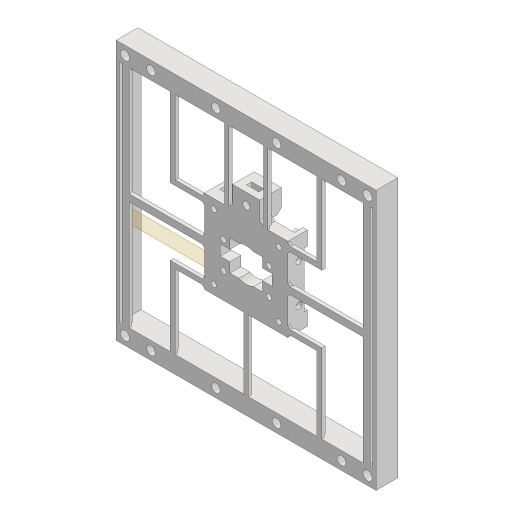
# Autodesk Inventor part: Flexible_cam_holder_v7_HQ
Saved by Autodesk Inventor 2023 (Build 270158000, 158)
## iProperties
Created: 2021-01-08
Part Number: Flexible_cam_holder_v7_HQ
Material: Generic
Document SubType Name: Sheet Metal
Designer: CDT
Density: 1 g/cm^3
Appearance: Default
Sheet Metal Rule: Default
Author: CDT
Autodesk Inventor part; units mm, degrees
ref_plane "YZ Plane" through (0, 0, 0) normal (1, 0, 0) x (0, 1, 0)
ref_plane "XZ Plane" through (0, 0, 0) normal (0, 1, 0) x (-1, 0, 0)
ref_plane "Work Plane1" through (0, 0, 0) normal (0, 0, 1) x (1, 0, 0)
sketch "Sketch1" plane through (0, 0, 0) normal (0, 0, 1) x (1, 0, 0)
  line L0 (-30.0874, -48.0547) -> (89.9126, -48.0547)
  line L1 (89.9126, -48.0547) -> (89.9126, 71.9453)
  line L2 (89.9126, 71.9453) -> (-30.0874, 71.9453)
  line L3 (-30.0874, 71.9453) -> (-30.0874, -48.0547)
  circle A0 centre (-26.0874, 67.9453) radius 2.125
  circle A1 centre (85.9126, 67.9453) radius 2.125
  circle A2 centre (85.9126, -44.0547) radius 2.125
  circle A3 centre (-26.0874, -44.0547) radius 2.125
  circle A4 centre (-14.0874, 67.9453) radius 2
  circle A5 centre (73.9126, 67.9453) radius 2
  circle A6 centre (-14.0874, -44.0547) radius 2
  circle A7 centre (73.9126, -44.0547) radius 2
  circle A8 centre (15.9126, 67.9453) radius 2
  circle A9 centre (43.9126, 67.9453) radius 2
  circle A10 centre (15.9126, -44.0547) radius 2
  circle A11 centre (43.9126, -44.0547) radius 2
  point P0 (0, 0)
  dimension "d0" = 120
  dimension "d1" = 120
  dimension "d2" = 4.25
  dimension "d3" = 4.25
  dimension "d4" = 4.25
  dimension "d5" = 4.25
  dimension "d107" = 4
  dimension "d108" = 4
  dimension "d109" = 4
  dimension "d110" = 4
  dimension "d111" = 4
  dimension "d112" = 4
  dimension "d113" = 4
  dimension "d114" = 4
  dimension "d172" = 4
  dimension "d173" = 4
  dimension "d174" = 4
  dimension "d175" = 4
  dimension "d176" = 16
  dimension "d177" = 4
  dimension "d178" = 4
  dimension "d179" = 16
  dimension "d180" = 16
  dimension "d181" = 4
  dimension "d182" = 4
  dimension "d183" = 16
  dimension "d729" = 4
  dimension "d730" = 4
  dimension "d731" = 4
  dimension "d732" = 4
  dimension "d733" = 4
  dimension "d734" = 4
  dimension "d735" = 4
  dimension "d736" = 4
  dimension "d737" = 46
  dimension "d738" = 46
  dimension "d739" = 46
  dimension "d740" = 46
  constraints: 12 centre point, 8 end point, 2 parallel, 1 horizontal, 1 perpendicular
  measures "d0" distance of L2.end L0.start
  measures "d1" distance of L1.end L2.end
  measures "d2" diameter of A0
  measures "d3" diameter of A1
  measures "d4" diameter of A2
  measures "d5" diameter of A3
  measures "d107" distance from line of L1 A1.centre
  measures "d108" distance from line of L3 A0.centre
  measures "d109" distance from line of L3 A3.centre
  measures "d110" distance from line of L1 A2.centre
  measures "d111" distance from line of L2 A0.centre
  measures "d112" distance from line of L2 A1.centre
  measures "d113" distance from line of L0 A2.centre
  measures "d114" distance from line of L0 A3.centre
  measures "d172" diameter of A4
  measures "d173" diameter of A5
  measures "d174" diameter of A6
  measures "d175" diameter of A7
  measures "d176" distance from line of A6.centre L3
  measures "d177" distance from line of L0 A6.centre
  measures "d178" distance from line of L0 A7.centre
  measures "d179" distance from line of L1 A7.centre
  measures "d180" distance from line of L1 A5.centre
  measures "d181" distance from line of L2 A5.centre
  measures "d182" distance from line of L2 A4.centre
  measures "d183" distance from line of L3 A4.centre
  measures "d729" diameter of A8
  measures "d730" diameter of A9
  measures "d731" diameter of A10
  measures "d732" diameter of A11
  measures "d733" distance from line of L2 A9.centre
  measures "d734" distance from line of L2 A8.centre
  measures "d735" distance from line of L0 A10.centre
  measures "d736" distance from line of L0 A11.centre
  measures "d737" distance from line of L1 A11.centre
  measures "d738" distance from line of L3 A10.centre
  measures "d739" distance from line of L3 A8.centre
  measures "d740" distance from line of L1 A9.centre
extrude "Extrusion1" add sketch "Sketch1" along normal blind 5
sketch "Sketch2" plane through (0, 0, 5) normal (0, 0, 1) x (1, 0, 0)
  line L0 (-24.0874, -40.0547) -> (10.6626, -40.0547)
  line L1 (10.6626, -40.0547) -> (10.6626, 10.3453)
  line L2 (10.6626, 10.3453) -> (-24.0874, 10.3453)
  line L3 (-24.0874, 10.3453) -> (-24.0874, -40.0547)
  line L4 (89.9126, -48.0547) -> (89.9126, 71.9453) projected
  line L5 (-30.0874, 71.9453) -> (-30.0874, -48.0547) projected
  line L6 (-30.0874, -48.0547) -> (89.9126, -48.0547) projected
  line L7 (89.9126, 71.9453) -> (-30.0874, 71.9453) projected
  line L8 (-24.0874, 13.5453) -> (10.6626, 13.5453)
  line L9 (10.6626, 13.5453) -> (10.6626, 63.9453)
  line L10 (10.6626, 63.9453) -> (-24.0874, 63.9453)
  line L11 (-24.0874, 63.9453) -> (-24.0874, 13.5453)
  line L12 (83.9126, -40.0547) -> (49.1626, -40.0547)
  line L13 (49.1626, -40.0547) -> (49.1626, 10.3453)
  line L14 (49.1626, 10.3453) -> (83.9126, 10.3453)
  line L15 (83.9126, 10.3453) -> (83.9126, -40.0547)
  line L16 (83.9126, 13.5453) -> (49.1626, 13.5453)
  line L17 (49.1626, 13.5453) -> (49.1626, 63.9453)
  line L18 (49.1626, 63.9453) -> (83.9126, 63.9453)
  line L19 (83.9126, 63.9453) -> (83.9126, 13.5453)
  line L20 (-24.0874, -40.0547) -> (83.9126, -40.0547)
  line L21 (83.9126, -40.0547) -> (83.9126, -7.3047)
  line L22 (83.9126, -7.3047) -> (-24.0874, -7.3047)
  line L23 (-24.0874, -7.3047) -> (-24.0874, -40.0547)
  line L24 (-24.0874, 63.9453) -> (83.9126, 63.9453)
  line L25 (83.9126, 63.9453) -> (83.9126, 31.1953)
  line L26 (83.9126, 31.1953) -> (-24.0874, 31.1953)
  line L27 (-24.0874, 31.1953) -> (-24.0874, 63.9453)
  line L28 (83.9126, 11.9453) -> (49.1626, 11.9453)
  line L29 (49.1626, 11.9453) -> (49.1626, 11.9453)
  line L30 (49.1626, 11.9453) -> (83.9126, 11.9453)
  line L31 (83.9126, 11.9453) -> (83.9126, 11.9453)
  line L32 (15.6626, 11.9453) -> (-24.0874, 11.9453)
  line L33 (-24.0874, 11.9453) -> (-24.0874, 11.9453)
  line L34 (-24.0874, 11.9453) -> (15.6626, 11.9453)
  line L35 (15.6626, 11.9453) -> (15.6626, 11.9453)
  line L36 (-27.3874, -40.0547) -> (-30.0874, -40.0547)
  line L37 (-30.0874, -40.0547) -> (-30.0874, 63.9453)
  line L38 (-30.0874, 63.9453) -> (-27.3874, 63.9453)
  line L39 (-27.3874, 63.9453) -> (-27.3874, -40.0547)
  line L40 (89.9126, 63.9453) -> (87.2126, 63.9453)
  line L41 (87.2126, 63.9453) -> (87.2126, -40.0547)
  line L42 (87.2126, -40.0547) -> (89.9126, -40.0547)
  line L43 (89.9126, -40.0547) -> (89.9126, 63.9453)
  line L44 (-30.0874, -48.0547) -> (-44.0088, -48.0547)
  line L45 (-44.0088, -48.0547) -> (-44.0088, 71.9453)
  line L46 (-44.0088, 71.9453) -> (-30.0874, 71.9453)
  line L47 (-30.0874, 71.9453) -> (-30.0874, -48.0547)
  point P0 (0, 0)
  point P1 (10.6626, 63.9453)
  point P2 (10.6626, 31.1953)
  point P3 (49.1626, 31.1953)
  point P4 (49.1626, -7.3047)
  point P5 (10.6626, -7.3047)
  point P6 (10.6626, -40.0547)
  point P7 (-30.0874, 63.9453)
  point P8 (-30.0874, -40.0547)
  point P9 (89.9126, -40.0547)
  dimension "d9" = 6
  dimension "d10" = 8
  dimension "d13" = 8
  dimension "d15" = 6
  dimension "d19" = 6
  dimension "d20" = 6
  dimension "d21" = 8
  dimension "d23" = 6
  dimension "d24" = 58.4
  dimension "d25" = 58.4
  dimension "d26" = 32.75
  dimension "d27" = 32.75
  dimension "d31" = 58.4
  dimension "d32" = 58.4
  dimension "d54" = 1.6
  dimension "d55" = 1.6
  dimension "d56" = 6
  dimension "d58" = 6
  dimension "d91" = 0
  dimension "d115" = 8
  dimension "d116" = 8
  dimension "d117" = 3.3
  dimension "d119" = 8
  dimension "d120" = 8
  dimension "d121" = 3.3
  dimension "d168" = 38.5
  dimension "d342" = 120
  dimension "d352" = 120
  dimension "d778" = 38.5
  dimension "d779" = 38.5
  dimension "d780" = 34.75
  dimension "d781" = 34.75
  constraints: 88 end point, 22 equal length, 11 horizontal, 11 perpendicular, 5 point on line, 3 collinear
  measures "d9" distance between parallel lines of L5 L3
  measures "d10" distance between parallel lines of L6 L0
  measures "d13" distance between parallel lines of L7 L10
  measures "d15" distance between parallel lines of L5 L11
  measures "d19" distance between parallel lines of L21 L4
  measures "d20" distance between parallel lines of L4 L15
  measures "d21" distance between parallel lines of L6 L12
  measures "d23" distance between parallel lines of L4 L19
  measures "d24" distance between parallel lines of L6 L14
  measures "d25" distance between parallel lines of L16 L7
  measures "d26" distance between parallel lines of L26 L24
  measures "d27" distance between parallel lines of L22 L20
  measures "d31" distance between parallel lines of L6 L2
  measures "d32" distance between parallel lines of L8 L7
  measures "d54" distance between parallel lines of L14 L28
  measures "d55" distance between parallel lines of L16 L30
  measures "d56" distance between parallel lines of L4 L31
  measures "d58" distance between parallel lines of L5 L33
  measures "d91" distance between parallel lines of L32 L34
  measures "d115" distance between parallel lines of L6 L36
  measures "d116" distance between parallel lines of L7 L38
  measures "d117" distance between parallel lines of L11 L39
  measures "d119" distance between parallel lines of L7 L40
  measures "d120" distance between parallel lines of L6 L42
  measures "d121" distance between parallel lines of L19 L41
  measures "d168" distance between parallel lines of L26 L22
  measures "d342" distance of L4.end L5.start
  measures "d352" distance of L44.end L45.end
  measures "d778" distance between parallel lines of L13 L1
  measures "d779" distance between parallel lines of L17 L9
  measures "d780" distance between parallel lines of L17 L19
  measures "d781" distance between parallel lines of L3 L1
extrude "Extrusion2" cut sketch "Sketch2" against normal blind 10 contours L3 L22 L1 L0 | L1 L22 L13 L20 | L3 L2 L1 L22 | L13 L22 L15 L12 | L13 L14 L15 L22 | L42 L41 L40 L4 | L5 L38 L39 L36 | L11 L26 L9 L8 | L11 L10 L9 L26 | L9 L24 L17 L26 | L26 L19 L16 L17 | L17 L18 L19 L26
sketch "Sketch3" plane through (0, 0, 5) normal (0, 0, 1) x (1, 0, 0)
  circle A0 centre (19.4126, 4.5953) radius 1.25
  circle A1 centre (19.4126, 17.0953) radius 1.25
  circle A2 centre (40.4126, 4.5953) radius 1.25
  circle A3 centre (40.4126, 17.0953) radius 1.25
  line L0 (49.1626, 31.1953) -> (10.6626, 31.1953) projected
  line L1 (10.6626, -7.3047) -> (49.1626, -7.3047) projected
  line L2 (49.1626, -7.3047) -> (49.1626, 10.3453) projected
  line L3 (10.6626, -7.3047) -> (10.6626, 10.3453) projected
  point P0 (0, 0)
  point P1 (36.9126, 39.9453)
  dimension "d257" = 2.5
  dimension "d258" = 2.5
  dimension "d259" = 2.5
  dimension "d260" = 2.5
  dimension "d261" = 12.5
  dimension "d262" = 12.5
  dimension "d263" = 21
  dimension "d264" = 21
  dimension "d265" = 0
  dimension "d266" = 0
  dimension "d455" = 38.5
  dimension "d456" = 38.5
  dimension "d457" = 11.9
  dimension "d458" = 11.9
  dimension "d459" = 8.75
  dimension "d741" = 8.75
  dimension "d759" = 14.1
  constraints: 4 centre point
  measures "d257" diameter of A0
  measures "d258" diameter of A1
  measures "d259" diameter of A2
  measures "d260" diameter of A3
  measures "d261" distance of A3.centre A2.centre
  measures "d262" distance of A1.centre A0.centre
  measures "d263" distance of A3.centre A1.centre
  measures "d264" distance of A2.centre A0.centre
  measures "d265" vertical distance of A2.centre A0.centre
  measures "d266" horizontal distance of A2.centre A3.centre
  measures "d455" distance between parallel lines of L0 L1
  measures "d456" distance of L1.start L1.end
  measures "d457" distance from line of A0.centre L1
  measures "d458" distance from line of L1 A2.centre
  measures "d459" distance from line of L2 A2.centre
  measures "d741" distance from line of L3 A0.centre
  measures "d759" distance from line of L0 A1.centre
ref_plane "Work Plane2" through (-30, 66, 0) normal (0, 0, 1) x (1, 0, 0)
extrude "Extrusion3" cut sketch "Sketch3" against normal up to surface (5 mm away)
sketch "Sketch34" plane through (0, 0, 5) normal (0, 0, 1) x (1, 0, 0)
  line L0 (-5.0874, 63.9453) -> (-2.7874, 63.9453)
  line L1 (-2.7874, 63.9453) -> (-2.7874, 27.4453)
  line L2 (-2.7874, 27.4453) -> (-5.0874, 27.4453)
  line L3 (-5.0874, 27.4453) -> (-5.0874, 63.9453)
  line L4 (-24.0874, 63.9453) -> (83.9126, 63.9453) projected
  line L5 (-24.0874, 13.5453) -> (-24.0874, 63.9453) projected
  line L6 (62.6126, 63.9453) -> (64.9126, 63.9453)
  line L7 (64.9126, 63.9453) -> (64.9126, 27.4453)
  line L8 (64.9126, 27.4453) -> (62.6126, 27.4453)
  line L9 (62.6126, 27.4453) -> (62.6126, 63.9453)
  line L10 (83.9126, 63.9453) -> (83.9126, 13.5453) projected
  line L11 (-2.7874, 27.4453) -> (10.6626, 27.4453)
  line L12 (10.6626, 27.4453) -> (10.6626, 29.7453)
  line L13 (10.6626, 29.7453) -> (-2.7874, 29.7453)
  line L14 (-2.7874, 29.7453) -> (-2.7874, 27.4453)
  line L15 (62.6126, 27.4453) -> (49.1626, 27.4453)
  line L16 (49.1626, 27.4453) -> (49.1626, 29.7453)
  line L17 (49.1626, 29.7453) -> (62.6126, 29.7453)
  line L18 (62.6126, 29.7453) -> (62.6126, 27.4453)
  line L19 (-5.0874, -40.0547) -> (-2.7874, -40.0547)
  line L20 (-2.7874, -40.0547) -> (-2.7874, -3.5547)
  line L21 (-2.7874, -3.5547) -> (-5.0874, -3.5547)
  line L22 (-5.0874, -3.5547) -> (-5.0874, -40.0547)
  line L23 (62.6126, -40.0547) -> (64.9126, -40.0547)
  line L24 (64.9126, -40.0547) -> (64.9126, -3.5547)
  line L25 (64.9126, -3.5547) -> (62.6126, -3.5547)
  line L26 (62.6126, -3.5547) -> (62.6126, -40.0547)
  line L27 (-24.0874, -40.0547) -> (-24.0874, 10.3453) projected
  line L28 (-2.7874, -3.5547) -> (10.6626, -3.5547)
  line L29 (10.6626, -3.5547) -> (10.6626, -5.8547)
  line L30 (10.6626, -5.8547) -> (-2.7874, -5.8547)
  line L31 (-2.7874, -5.8547) -> (-2.7874, -3.5547)
  line L32 (83.9126, 10.3453) -> (83.9126, -40.0547) projected
  line L33 (62.6126, -3.5547) -> (49.1626, -3.5547)
  line L34 (49.1626, -3.5547) -> (49.1626, -5.8547)
  line L35 (49.1626, -5.8547) -> (62.6126, -5.8547)
  line L36 (62.6126, -5.8547) -> (62.6126, -3.5547)
  line L37 (-30.0874, -48.0547) -> (89.9126, -48.0547) projected
  line L38 (89.9126, -48.0547) -> (-30.0874, -48.0547)
  line L39 (-30.0874, -48.0547) -> (-30.0874, -57.7562)
  line L40 (-30.0874, -57.7562) -> (89.9126, -57.7562)
  line L41 (89.9126, -57.7562) -> (89.9126, -48.0547)
  line L42 (-30.0874, 71.9453) -> (-30.0874, -48.0547) projected
  line L43 (-30.0874, -48.0547) -> (-47.0069, -48.0547)
  line L44 (-47.0069, -48.0547) -> (-47.0069, 71.9453)
  line L45 (-47.0069, 71.9453) -> (-30.0874, 71.9453)
  line L46 (-30.0874, 71.9453) -> (-30.0874, -48.0547)
  line L47 (-30.0874, 71.9453) -> (-30.0874, -48.0547) projected
  line L48 (89.9126, 71.9453) -> (-30.0874, 71.9453) projected
  line L49 (-22.0874, -40.0547) -> (81.9126, -40.0547) projected
  line L50 (49.1626, 31.1953) -> (49.1626, 13.5453) projected
  line L51 (49.1626, 10.3453) -> (49.1626, -7.3047) projected
  line L52 (10.6626, 10.3453) -> (10.6626, -7.3047) projected
  line L53 (10.6626, 31.1953) -> (10.6626, 13.5453) projected
  point P0 (-24.0874, 10.3453)
  point P1 (62.6126, -5.8547)
  point P2 (64.9126, 63.9453)
  point P3 (-2.7874, 29.7453)
  point P4 (-2.7874, -5.8547)
  point P5 (-30.0874, -40.0547)
  point P6 (99.9126, -40.0547)
  point P7 (54.1626, 36.1953)
  point P8 (83.9126, -40.0547)
  dimension "d317" = 0
  dimension "d318" = 36.5
  dimension "d319" = 19
  dimension "d320" = 2.3
  dimension "d321" = 2.3
  dimension "d322" = 36.5
  dimension "d323" = 0
  dimension "d324" = 19
  dimension "d326" = 2.3
  dimension "d328" = 2.3
  dimension "d329" = 19
  dimension "d330" = 2.3
  dimension "d333" = 2.3
  dimension "d335" = 19
  dimension "d336" = 2.3
  dimension "d337" = 36.5
  dimension "d339" = 2.3
  dimension "d364" = 120
  dimension "d365" = 120
  dimension "d373" = 36.5
  dimension "d374" = 36.5
  dimension "d782" = 0
  dimension "d783" = 0
  dimension "d785" = 0
  dimension "d786" = 0
  constraints: 80 end point, 20 parallel, 10 horizontal, 10 perpendicular, 2 collinear, 2 other
  measures "d317" distance between parallel lines of L4 L0
  measures "d318" distance between parallel lines of L2 L0
  measures "d319" distance between parallel lines of L3 L5
  measures "d320" distance between parallel lines of L1 L3
  measures "d321" distance of L7.end L8.end
  measures "d322" distance of L6.end L7.end
  measures "d323" distance between parallel lines of L4 L6
  measures "d324" distance between parallel lines of L10 L7
  measures "d326" distance of L12.end L11.end
  measures "d328" distance of L15.end L16.end
  measures "d330" distance between parallel lines of L20 L22
  measures "d333" distance of L28.end L29.end
  measures "d336" distance between parallel lines of L26 L24
  measures "d337" distance between parallel lines of L25 L23
  measures "d339" distance of L34.end L33.end
  measures "d364" distance of L42.start L37.start
  measures "d365" distance of L39.end L40.end
  measures "d373" distance between parallel lines of L49 L28
  measures "d374" distance between parallel lines of L49 L33
  measures "d782" distance between parallel lines of L50 L16
  measures "d783" distance between parallel lines of L51 L34
  measures "d785" distance between parallel lines of L52 L29
  measures "d786" distance between parallel lines of L53 L12
extrude "Extrusion32" add sketch "Sketch34" against normal blind 1.5 contours L0 L1 L2 L3 | L13 L12 L11 L1 | L4 L7 L8 L9 | L9 L15 L16 L17 | L22 L21 L20 L19 | L20 L28 L29 L30 | L26 L25 L24 L23 | L35 L34 L33 L26
chamfer "Chamfer5" distance 1 angle 45 12 edges at (49.1626, 10.3453, 2.5) (10.6626, 10.3453, 2.5) (10.6626, -5.8547, 4.25) (10.6626, -3.5547, 4.25) (49.1626, -3.5547, 4.25) (49.1626, -5.8547, 4.25) (49.1626, 13.5453, 2.5) (49.1626, 27.4453, 4.25) (49.1626, 29.7453, 4.25) (10.6626, 13.5453, 2.5) (10.6626, 27.4453, 4.25) (10.6626, 29.7453, 4.25)
sketch "Sketch38" plane through (0, 0, 0) normal (0, 0, -1) x (-1, 0, 0)
  line L0 (-89.9126, -48.0547) -> (30.0874, -48.0547)
  line L1 (30.0874, -48.0547) -> (30.0874, -40.0547)
  line L2 (30.0874, -40.0547) -> (-89.9126, -40.0547)
  line L3 (-89.9126, -40.0547) -> (-89.9126, -48.0547)
  circle A0 centre (-85.9126, -44.0547) radius 2.125 projected
  circle A1 centre (-85.9126, -44.0547) radius 2.125
  circle A2 centre (-73.9126, -44.0547) radius 2 projected
  circle A3 centre (-73.9126, -44.0547) radius 2
  circle A4 centre (14.0874, -44.0547) radius 2 projected
  circle A5 centre (14.0874, -44.0547) radius 2
  circle A6 centre (26.0874, -44.0547) radius 2.125 projected
  circle A7 centre (26.0874, -44.0547) radius 2.125
  circle A8 centre (26.0874, 67.9453) radius 2.125 projected
  circle A9 centre (26.0874, 67.9453) radius 2.125
  circle A10 centre (14.0874, 67.9453) radius 2 projected
  circle A11 centre (14.0874, 67.9453) radius 2
  circle A12 centre (-73.9126, 67.9453) radius 2 projected
  circle A13 centre (-73.9126, 67.9453) radius 2
  circle A14 centre (-85.9126, 67.9453) radius 2.125 projected
  circle A15 centre (-85.9126, 67.9453) radius 2.125
  circle A16 centre (-43.9126, -44.0547) radius 2 projected
  circle A17 centre (-43.9126, -44.0547) radius 2
  circle A18 centre (-15.9126, -44.0547) radius 2 projected
  circle A19 centre (-15.9126, -44.0547) radius 2
  circle A20 centre (-15.9126, 67.9453) radius 2 projected
  circle A21 centre (-15.9126, 67.9453) radius 2
  circle A22 centre (-43.9126, 67.9453) radius 2 projected
  circle A23 centre (-43.9126, 67.9453) radius 2
  line L4 (-89.9126, 63.9453) -> (-89.9126, 71.9453) projected
  line L5 (30.0874, 71.9453) -> (30.0874, 63.9453) projected
  line L6 (-89.9126, 71.9453) -> (30.0874, 71.9453)
  line L7 (30.0874, 71.9453) -> (30.0874, 63.9453)
  line L8 (30.0874, 63.9453) -> (-89.9126, 63.9453)
  line L9 (-89.9126, 63.9453) -> (-89.9126, 71.9453)
  constraints: 16 end point, 12 centre point, 12 coincident, 4 parallel, 2 horizontal, 2 perpendicular
extrude "Extrusion36" add sketch "Sketch38" along normal blind 5
sketch "Sketch43" plane through (0, 0, 5) normal (0, 0, 1) x (1, 0, 0)
  line L0 (30.9126, -40.0547) -> (28.9126, -40.0547)
  line L1 (28.9126, -40.0547) -> (28.9126, -7.3047)
  line L2 (28.9126, -7.3047) -> (30.9126, -7.3047)
  line L3 (30.9126, -7.3047) -> (30.9126, -40.0547)
  line L4 (21.9126, 31.1953) -> (19.9126, 31.1953)
  line L5 (19.9126, 31.1953) -> (19.9126, 63.9453)
  line L6 (19.9126, 63.9453) -> (21.9126, 63.9453)
  line L7 (21.9126, 63.9453) -> (21.9126, 31.1953)
  line L8 (-30.0874, 71.9453) -> (-30.0874, -48.0547) projected
  line L9 (-30.0874, 71.9453) -> (89.9126, 71.9453)
  line L10 (89.9126, 71.9453) -> (89.9126, 66.0007)
  line L11 (89.9126, 66.0007) -> (-30.0874, 66.0007)
  line L12 (-30.0874, 66.0007) -> (-30.0874, 71.9453)
  line L13 (-2.7874, 63.9453) -> (83.9126, 63.9453) projected
  line L14 (49.1626, 31.1953) -> (10.6626, 31.1953) projected
  line L15 (89.9126, -48.0547) -> (89.9126, 71.9453) projected
  line L16 (-30.0874, 71.9453) -> (-30.0874, -48.0547) projected
  line L17 (10.6626, -7.3047) -> (49.1626, -7.3047) projected
  line L18 (62.6126, -40.0547) -> (-2.7874, -40.0547) projected
  line L19 (37.9126, 31.1953) -> (39.9126, 31.1953)
  line L20 (39.9126, 31.1953) -> (39.9126, 63.9453)
  line L21 (39.9126, 63.9453) -> (37.9126, 63.9453)
  line L22 (37.9126, 63.9453) -> (37.9126, 31.1953)
  line L23 (89.9126, 71.9453) -> (-30.0874, 71.9453)
  line L24 (-30.0874, 71.9453) -> (-30.0874, 107.7464)
  line L25 (-30.0874, 107.7464) -> (89.9126, 107.7464)
  line L26 (89.9126, 107.7464) -> (89.9126, 71.9453)
  point P0 (0, 0)
  point P1 (62.6126, 63.9453)
  point P2 (47.1626, 36.1953)
  point P3 (22.6626, 36.1953)
  point P4 (-30.0874, -40.0547)
  point P5 (22.6626, -2.3047)
  point P6 (47.1626, -2.3047)
  point P7 (87.2126, 63.9453)
  point P8 (54.1626, 36.1953)
  point P9 (15.6626, 36.1953)
  point P10 (49.1626, -7.3047)
  point P11 (-25.3874, -40.0547)
  point P12 (10.6626, 31.1953)
  dimension "d442" = 50
  dimension "d444" = 2
  dimension "d445" = 0
  dimension "d446" = 0
  dimension "d448" = 59
  dimension "d449" = 2
  dimension "d450" = 0
  dimension "d451" = 0
  dimension "d774" = 50
  dimension "d775" = 2
  dimension "d776" = 0
  dimension "d806" = 0
  dimension "d808" = 120
  constraints: 40 end point, 10 parallel, 5 horizontal, 5 perpendicular, 2 other
  measures "d442" distance between parallel lines of L5 L8
  measures "d444" distance between parallel lines of L7 L5
  measures "d445" distance between parallel lines of L13 L6
  measures "d446" vertical extent of L4
  measures "d448" distance between parallel lines of L16 L1
  measures "d449" distance between parallel lines of L3 L1
  measures "d450" vertical extent of L2
  measures "d451" distance between parallel lines of L18 L0
  measures "d774" distance between parallel lines of L15 L20
  measures "d775" distance between parallel lines of L22 L20
  measures "d776" vertical extent of L19
  measures "d806" distance between parallel lines of L13 L21
  measures "d808" distance of L24.end L25.end
extrude "Extrusion41" add sketch "Sketch43" against normal up to surface (1.5 mm away) contours L0 L1 L2 L3 | L4 L5 L6 L7 | L22 L13 L20 L14
sketch "Sketch44" plane through (0, 0, 0) normal (0, 0, -1) x (-1, 0, 0)
  line L0 (-10.6626, -40.0547) -> (30.0874, -40.0547)
  line L1 (30.0874, -40.0547) -> (30.0874, 63.9453)
  line L2 (30.0874, 63.9453) -> (-10.6626, 63.9453)
  line L3 (-10.6626, 63.9453) -> (-10.6626, -40.0547)
  line L4 (-83.9126, 63.9453) -> (24.0874, 63.9453) projected
  line L5 (-10.6626, 13.5453) -> (-10.6626, 31.1953) projected
  line L6 (24.0874, -40.0547) -> (-83.9126, -40.0547) projected
  line L7 (30.0874, -40.0547) -> (30.0874, -48.0547) projected
  line L8 (-49.1626, -40.0547) -> (-89.9126, -40.0547)
  line L9 (-89.9126, -40.0547) -> (-89.9126, 63.9453)
  line L10 (-89.9126, 63.9453) -> (-49.1626, 63.9453)
  line L11 (-49.1626, 63.9453) -> (-49.1626, -40.0547)
  line L12 (-89.9126, -48.0547) -> (-89.9126, -40.0547) projected
  line L13 (-49.1626, 10.3453) -> (-49.1626, -7.3047) projected
  point P0 (0, 0)
  point P1 (-83.9126, -40.0547)
  point P2 (-49.1626, -40.0547)
  point P3 (-49.1626, 63.9453)
  dimension "d464" = 0
  dimension "d465" = 0
  dimension "d466" = 0
  dimension "d467" = 0
  dimension "d468" = 0
  dimension "d469" = 0
  dimension "d470" = 0
  dimension "d471" = 0
  constraints: 16 end point, 4 parallel, 2 horizontal, 2 perpendicular
  measures "d464" distance between parallel lines of L4 L2
  measures "d465" distance between parallel lines of L5 L3
  measures "d466" distance between parallel lines of L6 L0
  measures "d467" distance between parallel lines of L7 L1
  measures "d468" distance between parallel lines of L6 L8
  measures "d469" distance between parallel lines of L12 L9
  measures "d470" distance between parallel lines of L13 L11
  measures "d471" distance between parallel lines of L4 L10
extrude "Extrusion42" cut sketch "Sketch44" against normal blind 3.4 contours L3 L2 L1 L0 | L6 L8 L9 L10 L4 L11
sketch "Sketch45" plane through (0, 0, 0) normal (0, 0, -1) x (-1, 0, 0)
  circle A0 centre (-44.9126, -3.0547) radius 1.25
  circle A1 centre (-44.9126, 26.9453) radius 1.25
  circle A2 centre (-14.9126, -3.0547) radius 1.25
  circle A3 centre (-14.9126, 26.9453) radius 1.25
  line L0 (-49.1626, -7.3047) -> (-49.1626, 10.3453) projected
  line L1 (-37.9126, 31.1953) -> (-21.9126, 31.1953) projected
  line L2 (-49.1626, -7.3047) -> (-10.6626, -7.3047)
  line L3 (-10.6626, -7.3047) -> (-10.6626, 31.1953)
  line L4 (-10.6626, 31.1953) -> (-49.1626, 31.1953)
  line L5 (-49.1626, 31.1953) -> (-49.1626, -7.3047)
  point P0 (0, 0)
  point P1 (-53.4126, 15.3453)
  point P2 (-49.1626, 31.1953)
  point P3 (-53.4126, 26.9453)
  point P4 (-54.1626, 23.9453)
  point P5 (-54.1626, 21.5453)
  point P6 (-47.1626, 36.1953)
  point P7 (-22.6626, 36.1953)
  point P8 (-54.1626, -8.3047)
  point P9 (-19.9126, 31.1953)
  point P10 (-49.1626, 16.9453)
  point P11 (-49.1626, -6.8547)
  point P12 (-49.1626, 10.3453)
  point P13 (-21.9126, 31.1953)
  dimension "d474" = 2.5
  dimension "d475" = 2.5
  dimension "d476" = 2.5
  dimension "d477" = 2.5
  dimension "d478" = 30
  dimension "d479" = 30
  dimension "d480" = 30
  dimension "d481" = 30
  dimension "d482" = 4.25
  dimension "d483" = 38.5
  dimension "d484" = 4.25
  dimension "d485" = 4.25
  dimension "d486" = 4.25
  constraints: 6 end point, 4 centre point, 1 horizontal, 1 parallel, 1 perpendicular, 1 vertical, 5 other
  measures "d474" diameter of A0
  measures "d475" diameter of A1
  measures "d476" diameter of A2
  measures "d477" diameter of A3
  measures "d478" distance of A1.centre A0.centre
  measures "d479" distance of A3.centre A1.centre
  measures "d480" distance of A2.centre A0.centre
  measures "d481" distance of A3.centre A2.centre
  measures "d482" distance from line of L2 A0.centre
  measures "d483" distance of L2.end L3.end
  measures "d484" distance from line of L2 A2.centre
extrude "Extrusion43" cut sketch "Sketch45" against normal blind 7 contours A0 | A1 | A2 | A3
sketch "Sketch56" plane through (0, 0, -5) normal (0, 0, -1) x (-1, 0, 0)
  line L0 (30.0874, 63.9453) -> (28.5874, 63.9453)
  line L1 (28.5874, 63.9453) -> (28.5874, -40.0547)
  line L2 (28.5874, -40.0547) -> (30.0874, -40.0547)
  line L3 (30.0874, -40.0547) -> (30.0874, 63.9453)
  line L4 (-89.9126, 63.9453) -> (-88.4126, 63.9453)
  line L5 (-88.4126, 63.9453) -> (-88.4126, -40.0547)
  line L6 (-88.4126, -40.0547) -> (-89.9126, -40.0547)
  line L7 (-89.9126, -40.0547) -> (-89.9126, 63.9453)
  line L8 (30.0874, -40.0547) -> (-89.9126, -40.0547) projected
  point P0 (0, 0)
  dimension "d655" = 1.5
  dimension "d656" = 1.5
  dimension "d807" = 0
  constraints: 16 end point, 4 parallel, 2 horizontal, 2 perpendicular, 1 point on line
  measures "d655" distance of L2.end L1.end
  measures "d656" distance of L5.end L6.end
  measures "d807" distance between parallel lines of L8 L6
extrude "Extrusion54" add sketch "Sketch56" against normal up to surface (10 mm away)
sketch "Sketch60" plane through (0, 0, 0) normal (0, 0, -1) x (-1, 0, 0)
  line L0 (-10.6626, -6.8547) -> (-10.6626, -7.3047) projected
  line L1 (-10.6626, -7.3047) -> (-49.1626, -7.3047)
  line L2 (-49.1626, -7.3047) -> (-49.1626, -15.3047)
  line L3 (-10.6626, -15.3047) -> (-10.6626, -7.3047)
  line L4 (-10.6626, -7.3047) -> (-12.6626, -7.3047)
  line L5 (-12.6626, -7.3047) -> (-12.6626, 31.1953)
  line L6 (-12.6626, 31.1953) -> (-10.6626, 31.1953)
  line L7 (-10.6626, 31.1953) -> (-10.6626, -7.3047)
  line L8 (-49.1626, -7.3047) -> (-49.1626, 9.3453) projected
  line L9 (-49.1626, -7.3047) -> (-47.1626, -7.3047)
  line L10 (-47.1626, -7.3047) -> (-47.1626, 31.1953)
  line L11 (-47.1626, 31.1953) -> (-49.1626, 31.1953)
  line L12 (-49.1626, 31.1953) -> (-49.1626, -7.3047)
  circle A0 centre (-14.9126, 26.9453) radius 1.25 projected
  circle A1 centre (-14.9126, 26.9453) radius 2.4
  circle A2 centre (-14.9126, 26.9453) radius 1.25
  circle A3 centre (-14.9126, -3.0547) radius 1.25 projected
  circle A4 centre (-14.9126, -3.0547) radius 1.3
  circle A5 centre (-14.9126, -3.0547) radius 2.4
  circle A6 centre (-44.9126, -3.0547) radius 1.25 projected
  circle A7 centre (-44.9126, -3.0547) radius 1.3
  circle A8 centre (-44.9126, -3.0547) radius 2.4
  circle A9 centre (-44.9126, 26.9453) radius 1.25 projected
  circle A10 centre (-44.9126, 26.9453) radius 1.3
  circle A11 centre (-44.9126, 26.9453) radius 2.4
  point P0 (0, 0)
  point P1 (-15.6626, 36.1953)
  point P2 (-54.1626, 36.1953)
  point P3 (-47.1626, -3.8898)
  point P4 (-15.6626, 36.1953)
  point P5 (-12.6626, 27.7805)
  point P6 (-12.6626, 26.1102)
  point P7 (-12.6626, -2.2195)
  point P8 (-47.1626, -2.2195)
  point P9 (-47.1626, 26.1102)
  point P10 (-47.1626, 27.7805)
  point P11 (-54.1626, 36.1953)
  point P12 (-12.6626, -7.3047)
  point P13 (-47.1626, -7.3047)
  point P14 (-10.6626, 9.3453)
  point P15 (-49.1626, 9.3453)
  point P16 (-49.1626, 9.3453)
  point P17 (-10.6626, 10.3453)
  point P18 (-49.1626, 10.3453)
  point P19 (-12.6626, -1.5047)
  point P20 (-10.6626, 1.0453)
  point P21 (-49.1626, 29.2996)
  point P22 (-49.1626, 34.5911)
  point P23 (-49.1626, -0.7004)
  point P24 (-49.1626, 4.5911)
  point P25 (-49.1626, 12.3453)
  point P26 (-10.6626, 4.0453)
  point P27 (-49.1626, 9.3453)
  point P28 (-12.6626, -3.8898)
  dimension "d682" = 2
  dimension "d683" = 38.5
  dimension "d684" = 2
  dimension "d685" = 38.5
  dimension "d686" = 4.8
  dimension "d687" = 4.8
  dimension "d688" = 4.8
  dimension "d689" = 4.8
  constraints: 22 end point, 8 centre point, 8 coincident, 5 parallel, 3 horizontal, 3 perpendicular, 1 concentric, 2 other
  measures "d682" distance of L5.end L6.end
  measures "d683" distance of L4.end L5.end
  measures "d684" distance of L11.end L10.end
  measures "d685" distance of L10.end L9.end
  measures "d686" diameter of A1
  measures "d687" diameter of A5
  measures "d688" diameter of A8
  measures "d689" diameter of A11
extrude "Extrusion58" add sketch "Sketch60" along normal blind 4 contours L0 L1 L5 A5 A1 L6 L7 | A5 L5 | L5 A5 | A1 L5 | L5 A1 | L1 L8 L12 L11 L10 A11 A8 | A8 L10 | L10 A8 | A11 L10 | L10 A11 | A4 | A7 | A10
chamfer "Chamfer9" distance 3.5 angle 45 1 edges at (29.9126, -7.3047, 0)
sketch "Sketch61" plane through (0, 0, 5) normal (0, 0, 1) x (1, 0, 0)
  line L0 (23.6626, 31.1953) -> (36.1626, 31.1953)
  line L1 (36.1626, 31.1953) -> (36.1626, 41.1953)
  line L2 (36.1626, 41.1953) -> (23.6626, 41.1953)
  line L3 (23.6626, 41.1953) -> (23.6626, 31.1953)
  circle A0 centre (29.9126, 35.9453) radius 1.65
  line L4 (-30.0874, 71.9453) -> (-30.0874, -48.0547) projected
  line L5 (89.9126, 71.9453) -> (-30.0874, 71.9453) projected
  line L6 (-30.0874, -48.0547) -> (89.9126, -48.0547)
  line L7 (89.9126, -48.0547) -> (89.9126, 71.9453)
  line L8 (89.9126, 71.9453) -> (-30.0874, 71.9453)
  line L9 (-30.0874, 71.9453) -> (-30.0874, -48.0547)
  line L10 (49.1626, 31.1953) -> (10.6626, 31.1953) projected
  line L11 (49.1626, -7.3047) -> (49.1626, 9.3453) projected
  line L12 (10.6626, -6.8547) -> (10.6626, -7.3047) projected
  point P0 (0, 0)
  point P1 (54.1626, 36.1953)
  point P2 (15.6626, 36.1953)
  point P3 (49.1626, 9.3453)
  point P4 (10.6626, 9.3453)
  point P5 (49.1626, 10.3453)
  point P6 (10.6626, 10.3453)
  point P7 (10.6626, 31.1953)
  point P8 (10.6626, 4.0453)
  dimension "d695" = 3.3
  dimension "d696" = 60
  dimension "d697" = 120
  dimension "d698" = 84
  dimension "d699" = 0
  dimension "d700" = 13
  dimension "d701" = 13
  dimension "d702" = 10
  constraints: 16 end point, 4 parallel, 2 horizontal, 2 perpendicular, 1 centre point, 3 other
  measures "d695" diameter of A0
  measures "d696" distance from line of L4 A0.centre
  measures "d697" distance of L5.start L4.start
  measures "d698" distance from line of L6 A0.centre
  measures "d699" vertical extent of L0
  measures "d702" distance between parallel lines of L0 L2
extrude "Extrusion59" add sketch "Sketch61" against normal blind 10 contours L3 L2 L1 L0
chamfer "Chamfer10" distance 2 angle 45 1 edges at (29.9126, 31.1953, -5)
sketch "Sketch62" plane through (23.6626, 41.1953, 5) normal (0, 1, 0) x (1, 0, 0)
  line L0 (3.4, 5.4) -> (9.1, 5.4)
  line L1 (9.1, 5.4) -> (9.1, 3)
  line L2 (9.1, 3) -> (3.4, 3)
  line L3 (3.4, 3) -> (3.4, 5.4)
  line L4 (0, 0) -> (0, 10) projected
  line L5 (12.5, 0) -> (12.5, 10) projected
  line L6 (12.5, 0) -> (0, 0) projected
  point P0 (-23.6626, 5)
  dimension "d709" = 5.7
  dimension "d710" = 2.4
  dimension "d711" = 3.4
  dimension "d712" = 3.4
  dimension "d830" = 3
  constraints: 8 end point, 2 parallel, 1 horizontal, 1 perpendicular
  measures "d709" distance between parallel lines of L1 L3
  measures "d710" distance between parallel lines of L0 L2
  measures "d711" distance between parallel lines of L4 L3
  measures "d712" distance between parallel lines of L5 L1
  measures "d830" distance between parallel lines of L6 L2
extrude "Extrusion60" cut sketch "Sketch62" against normal blind 11
sketch "Sketch63" plane through (49.1626, -7.3047, 5) normal (1, 0, 0) x (0, 0, -1)
  circle A0 centre (5.2, 28.25) radius 1.5
  circle A1 centre (5.2, 10.25) radius 1.5
  line L0 (0, 0) -> (0, 16.65) projected
  line L1 (0, 38.5) -> (5, 38.5) projected
  line L2 (0, 0) -> (5, 0) projected
  point P0 (5, 7.3047)
  point P1 (9, 38.5)
  point P2 (9, 0)
  point P3 (0, 17.65)
  dimension "d718" = 3
  dimension "d719" = 3
  dimension "d720" = 5.2
  dimension "d721" = 5.2
  dimension "d722" = 10.25
  dimension "d723" = 10.25
  constraints: 2 centre point
  measures "d718" diameter of A0
  measures "d719" diameter of A1
  measures "d720" distance from line of L0 A1.centre
  measures "d721" distance from line of L0 A0.centre
  measures "d722" distance from line of L1 A0.centre
  measures "d723" distance from line of L2 A1.centre
extrude "Extrusion61" cut sketch "Sketch63" against normal blind 5
chamfer "Chamfer11" distance 2 angle 45 2 edges at (23.6626, 31.1953, 2.5) (36.1626, 31.1953, 2.5)
sketch "Sketch65" plane through (0, 0, 0) normal (0, 0, -1) x (-1, 0, 0)
  line L0 (-17.6626, 0.6953) -> (-42.1626, 0.6953)
  line L1 (-42.1626, 0.6953) -> (-42.1626, -7.3047)
  line L2 (-42.1626, -7.3047) -> (-17.6626, -7.3047)
  line L3 (-17.6626, -7.3047) -> (-17.6626, 0.6953)
  line L4 (-49.1626, -7.3047) -> (-12.6626, -7.3047) projected
  line L5 (-12.6626, 26.1102) -> (-12.6626, -2.2195) projected
  line L6 (-49.1626, 31.1953) -> (-49.1626, -7.3047) projected
  line L7 (-47.1626, -7.3047) -> (-47.1626, 31.1953) projected
  point P0 (0, 0)
  point P1 (-47.1626, -7.3047)
  point P2 (-47.1626, -3.8898)
  point P3 (-10.6626, -7.3047)
  dimension "d752" = 0
  dimension "d753" = 5
  dimension "d755" = 5
  dimension "d756" = 8
  constraints: 8 end point, 2 parallel, 1 horizontal, 1 perpendicular
  measures "d752" distance between parallel lines of L4 L2
  measures "d753" distance between parallel lines of L5 L3
  measures "d755" distance between parallel lines of L7 L1
  measures "d756" distance between parallel lines of L2 L0
extrude "Extrusion63" cut sketch "Sketch65" against normal blind 2.75
sketch "Sketch66" plane through (0, 0, 5) normal (0, 0, 1) x (1, 0, 0)
  circle A0 centre (29.9126, 12.0953) radius 7.75
  circle A1 centre (40.4126, 17.0953) radius 1.25 projected
  line L0 (41.9126, 14.5953) -> (17.9126, 14.5953)
  line L1 (17.9126, 14.5953) -> (17.9126, 9.5953)
  line L2 (17.9126, 9.5953) -> (41.9126, 9.5953)
  line L3 (41.9126, 9.5953) -> (41.9126, 14.5953)
  circle A2 centre (40.4126, 4.5953) radius 1.25 projected
  line L4 (10.6626, 31.1953) -> (10.6626, -7.3047) projected
  line L5 (49.1626, -7.3047) -> (49.1626, 31.1953) projected
  line L6 (37.4126, 19.0953) -> (22.4126, 19.0953)
  line L7 (22.4126, 19.0953) -> (22.4126, 5.0953)
  line L8 (22.4126, 5.0953) -> (37.4126, 5.0953)
  line L9 (37.4126, 5.0953) -> (37.4126, 19.0953)
  point P0 (0, 0)
  point P1 (22.5769, 9.5953)
  point P2 (37.2483, 9.5953)
  point P3 (37.2483, 14.5953)
  point P4 (22.5769, 14.5953)
  point P5 (37.4126, 9.5953)
  point P6 (22.4126, 9.5953)
  point P7 (22.4126, 14.5953)
  point P8 (37.4126, 14.5953)
  point P9 (33.2386, 5.0953)
  point P10 (33.2386, 19.0953)
  point P11 (26.5865, 5.0953)
  point P12 (26.5865, 19.0953)
  point P13 (22.4126, 10.1428)
  point P14 (22.4126, 14.0479)
  point P15 (37.4126, 10.1428)
  point P16 (37.4126, 14.0479)
  point P17 (10.6626, 4.0453)
  point P18 (49.1626, 15.3453)
  point P19 (10.6626, -6.8547)
  point P20 (49.1626, 9.3453)
  dimension "d760" = 15.5
  dimension "d761" = 5
  dimension "d762" = 2.5
  dimension "d763" = 5
  dimension "d764" = 12
  dimension "d765" = 12
  dimension "d766" = 19.25
  dimension "d767" = 19.25
  dimension "d770" = 7
  dimension "d771" = 7.5
  dimension "d772" = 7
  dimension "d773" = 7.5
  constraints: 16 end point, 4 parallel, 2 horizontal, 2 perpendicular, 1 centre point
  measures "d760" diameter of A0
  measures "d761" vertical distance of A0.centre A1.centre
  measures "d762" distance from line of A1.centre L0
  measures "d763" distance from line of A2.centre L2
  measures "d764" distance from line of A0.centre L3
  measures "d765" distance from line of L1 A0.centre
  measures "d766" distance from line of L4 A0.centre
  measures "d767" distance from line of L5 A0.centre
  measures "d770" distance from line of A0.centre L6
  measures "d771" distance from line of L9 A0.centre
  measures "d772" distance from line of L8 A0.centre
  measures "d773" distance from line of L7 A0.centre
extrude "Extrusion64" cut sketch "Sketch66" against normal up to surface (5 mm away) contours A0 L9 | A0 L9 L0 L3 L2 | L9 A0 L2 L7 L0 | A0 L0 L9 | L9 L2 A0 | L0 A0 L6 | A0 L6 L9 L0 | L2 L9 L8 A0 | A0 L8 L2 | L6 A0 | L0 L7 L6 A0 | A0 L7 L0 | A0 L8 | L2 L7 A0 | A0 L8 L7 L2 | L7 A0 | A0 L7 L2 L1 L0
sketch "Sketch67" plane through (0, 0, 3.5) normal (0, 0, -1) x (-1, 0, 0)
  line L0 (27.3874, 63.9453) -> (27.3874, -40.0547) projected
  line L1 (-87.2126, -40.0547) -> (-87.2126, 63.9453) projected
  line L2 (27.3874, 63.9453) -> (-87.2126, 63.9453)
  line L3 (-87.2126, 63.9453) -> (-87.2126, 62.4453)
  line L4 (-87.2126, 62.4453) -> (27.3874, 62.4453)
  line L5 (27.3874, 62.4453) -> (27.3874, 63.9453)
  line L6 (-87.2126, -40.0547) -> (27.3874, -40.0547)
  line L7 (27.3874, -40.0547) -> (27.3874, -38.5547)
  line L8 (27.3874, -38.5547) -> (-87.2126, -38.5547)
  line L9 (-87.2126, -38.5547) -> (-87.2126, -40.0547)
  line L10 (-49.1626, -7.3047) -> (-49.1626, -6.8547) projected
  line L11 (-49.1626, -7.3047) -> (-50.6626, -7.3047)
  line L12 (-50.6626, -7.3047) -> (-50.6626, 31.1953)
  line L13 (-50.6626, 31.1953) -> (-49.1626, 31.1953)
  line L14 (-49.1626, 31.1953) -> (-49.1626, -7.3047)
  line L15 (-39.9126, 31.1953) -> (-39.9126, 63.9453) projected
  line L16 (-37.9126, 63.9453) -> (-37.9126, 31.4453) projected
  line L17 (-39.9126, 31.1953) -> (-37.9126, 31.1953)
  line L18 (-37.9126, 31.1953) -> (-37.9126, 32.1953)
  line L19 (-37.9126, 32.1953) -> (-39.9126, 32.1953)
  line L20 (-39.9126, 32.1953) -> (-39.9126, 31.1953)
  line L21 (-19.9126, 63.9453) -> (-19.9126, 31.1953) projected
  line L22 (-19.9126, 31.1953) -> (-21.9126, 31.1953)
  line L23 (-21.9126, 31.1953) -> (-21.9126, 32.1953)
  line L24 (-21.9126, 32.1953) -> (-19.9126, 32.1953)
  line L25 (-19.9126, 32.1953) -> (-19.9126, 31.1953)
  line L26 (-10.6626, 31.1953) -> (-9.1626, 31.1953)
  line L27 (-9.1626, 31.1953) -> (-9.1626, -7.3047)
  line L28 (-9.1626, -7.3047) -> (-10.6626, -7.3047)
  line L29 (-10.6626, -7.3047) -> (-10.6626, 31.1953)
  line L30 (-28.9126, -7.3047) -> (-28.9126, -40.0547) projected
  line L31 (-30.9126, -40.0547) -> (-30.9126, -7.3047) projected
  line L32 (-28.9126, -7.3047) -> (-30.9126, -7.3047)
  line L33 (-30.9126, -7.3047) -> (-30.9126, -8.3047)
  line L34 (-30.9126, -8.3047) -> (-28.9126, -8.3047)
  line L35 (-28.9126, -8.3047) -> (-28.9126, -7.3047)
  point P0 (0, 0)
  point P1 (-30.9126, -7.3047)
  point P2 (-30.9126, -38.5547)
  point P3 (-28.9126, -38.5547)
  point P4 (27.3874, -38.5547)
  point P5 (-37.9126, 31.4453)
  point P6 (-87.2126, 63.9453)
  point P7 (27.3874, 62.4453)
  dimension "d812" = 1.5
  dimension "d813" = 1.5
  dimension "d814" = 1.5
  dimension "d815" = 1
  dimension "d816" = 2
  dimension "d817" = 1
  dimension "d818" = 1.5
  dimension "d819" = 1
  constraints: 56 end point, 14 parallel, 7 horizontal, 7 perpendicular, 4 point on line
  measures "d812" distance of L3.end L2.end
  measures "d813" distance of L7.end L6.end
  measures "d814" distance of L12.end L13.end
  measures "d815" distance of L18.end L17.end
  measures "d816" distance of L23.end L24.end
  measures "d817" distance of L22.end L23.end
  measures "d818" distance of L27.end L28.end
  measures "d819" distance of L33.end L32.end
extrude "Extrusion65" cut sketch "Sketch67" along normal mid plane 1 contours L0 L4 L21 L2 | L21 L4 L16 L2 | L0 L6 L30 L8 | L16 L4 L15 L2 | L15 L4 L1 L2 | L31 L6 L1 L8 | L34 L31 L32 L30 | L16 L18 L17 L15 L19 | L11 L12 L13 L14 L10 | L21 L22 L23 L24 | L26 L27 L28 L29
sketch "Sketch68" plane through (0, 0, -4) normal (0, 0, -1) x (-1, 0, 0)
  line L0 (-10.6626, -0.8047) -> (-49.1626, -0.8047)
  line L1 (-49.1626, -0.8047) -> (-49.1626, 24.6953)
  line L2 (-49.1626, 24.6953) -> (-10.6626, 24.6953)
  line L3 (-10.6626, 24.6953) -> (-10.6626, -0.8047)
  line L4 (-10.6626, 31.1953) -> (-12.6626, 31.1953) projected
  line L5 (-47.1626, -7.3047) -> (-12.6626, -7.3047) projected
  line L6 (-10.6626, -7.3047) -> (-10.6626, 31.1953) projected
  line L7 (-49.1626, 31.1953) -> (-49.1626, -7.3047) projected
  point P0 (0, 0)
  dimension "d822" = 6.5
  dimension "d823" = 6.5
  dimension "d824" = 0
  dimension "d825" = 0
  constraints: 8 end point, 2 parallel, 1 horizontal, 1 perpendicular
  measures "d822" distance between parallel lines of L4 L2
  measures "d823" distance between parallel lines of L5 L0
  measures "d824" distance between parallel lines of L6 L3
  measures "d825" distance between parallel lines of L7 L1
extrude "Extrusion66" cut sketch "Sketch68" against normal blind 1.5
sketch "Sketch69" plane through (10.6626, -2.5547, 5) normal (-1, 0, 0) x (0, 0, 1)
  arc A0 (-5, 24.9866) -> (-5, 22.0134) centre (-5.2, 23.5) ccw projected
  circle A1 centre (-5.2, 23.5) radius 1.5
  circle A2 centre (-5.2, 5.5) radius 1.5 projected
  circle A3 centre (-5.2, 5.5) radius 1.5
  point P0 (-5, 2.5547)
  point P1 (-5, 22.0134)
  point P2 (-5, 24.9866)
  constraints: 2 centre point, 2 coincident
extrude "Extrusion67" cut sketch "Sketch69" against normal blind 5
sketch "Sketch70" plane through (0, 0, -5) normal (0, 0, -1) x (-1, 0, 0)
  circle A0 centre (-29.9126, 35.9453) radius 1.65 projected
  circle A1 centre (-29.9126, 35.9453) radius 2.75
  circle A2 centre (-29.9126, 35.9453) radius 1.65
  point P0 (0, 0)
  dimension "d831" = 5.5
  dimension "d832" = 3.3
  constraints: 2 centre point, 2 coincident
  measures "d831" diameter of A1
  measures "d832" diameter of A2
extrude "Extrusion68" add sketch "Sketch70" along normal blind 2
equation "\"d9\" = d15"
equation "\"d19\" = d56"
equation "\"d20\" = d56"
equation "\"d23\" = d56"
equation "\"d24\" = d32"
equation "\"d25\" = d32"
equation "\"d31\" = d32"
equation "\"d58\" = d15"
body "Solid1"
